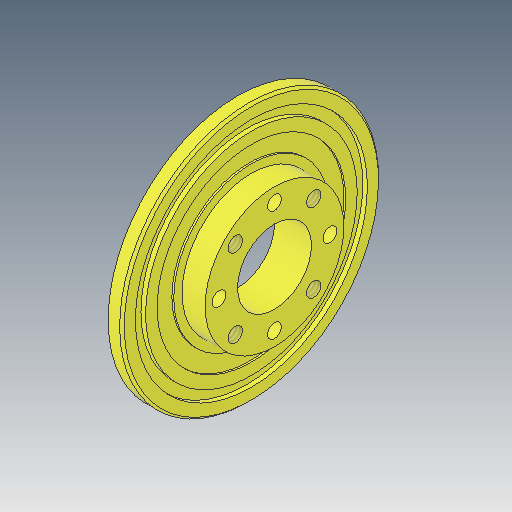
# Autodesk Inventor part: COXA_PITCH_BEARING_BASE
Saved by Autodesk Inventor 2019.4 (Build 234330000, 330)
## iProperties
Created: 2019-11-12
Part Number: COXA_PITCH_BEARING_BASE
Material: 一般
Document SubType Name: Modeling
Designer: y6tada
Density: 1 g/cm^3
Appearance: 滑らか - 黄
Mass: 1.03998 g
Surface Area: 16.9167 cm^2
Volume: 1.03998 cm^3
Author: y6tada
Autodesk Inventor part; units mm, degrees
ref_plane "YZ Plane" through (0, 0, 0) normal (1, 0, 0) x (0, 1, 0)
ref_plane "XZ Plane" through (0, 0, 0) normal (0, 1, 0) x (-1, 0, 0)
ref_plane "XY Plane" through (0, 0, 0) normal (0, 0, 1) x (1, 0, 0)
sketch "スケッチ1" plane through (0, 0, 0) normal (1, 0, 0) x (0, 1, 0)
  circle A0 centre (0, 0) radius 14
  circle A1 centre (0, 0) radius 4
  dimension "d0" = 8
  dimension "d1" = 28
  constraints: 2 centre point, 2 coincident
  measures "d0" diameter of A1
  measures "d1" diameter of A0
extrude "押し出し1" add sketch "スケッチ1" along normal blind 1.5
sketch "スケッチ2" plane through (1.5, 0, 0) normal (1, 0, 0) x (0, 0, -1)
  circle A0 centre (0, 0) radius 4 projected
  circle A1 centre (0, 0) radius 7.5
  dimension "d9" = 15
  constraints: 1 centre point, 1 coincident
  measures "d9" diameter of A1
extrude "押し出し2" add sketch "スケッチ2" along normal blind 2.5
sketch "スケッチ3" plane through (4, 0, 0) normal (1, 0, 0) x (0, 0, -1)
  circle A0 centre (0, 0) radius 6 construction
  line L0 (0, 0) -> (6, 0) construction
  point P0 (0, 6)
  point P1 (-6, 0)
  point P2 (0, -6)
  dimension "d12" = 12
  dimension "d15" = 360
  constraints: 2 end point, 1 coincident, 1 horizontal, 1 horizontal alignment, 7 other
hole "穴1" at (4, 0, -6) at (4, 6, 0) at (4, 0, 6) at (4, -6, 0) direction (-1, 0, 0) diameter 1.5 end through all both
sketch "スケッチ4" plane through (4, 0, 0) normal (1, 0, 0) x (0, 0, -1)
  line L0 (0, 0) -> (4.2426, 4.2426) construction
  circle A0 centre (0, 0) radius 6 construction
  line L1 (0, 0) -> (12.9289, 0) construction
  point P0 (-4.2426, 4.2426)
  point P1 (-4.2426, -4.2426)
  point P2 (4.2426, -4.2426)
  dimension "d25" = 12
  dimension "d24" = 45
  dimension "d28" = 360
  constraints: 4 end point, 1 coincident, 1 horizontal, 8 other
  measures "d24" angle of L1 L0
hole "穴2" at (4, 4.2426, -4.2426) at (4, 4.2426, 4.2426) at (4, -4.2426, 4.2426) at (4, -4.2426, -4.2426) direction (-1, 0, 0) diameter 1.567 end through all thread size "M2x0.4" class "6H" standard "ISO Metric profile"
sketch "スケッチ7" plane through (1.5, 0, 0) normal (1, 0, 0) x (0, 0, -1)
  circle A0 centre (0, 0) radius 8.4
  circle A1 centre (0, 0) radius 10.2
  dimension "d37" = 16.8
  dimension "d48" = 20.4
  constraints: 2 centre point, 2 coincident
  measures "d37" diameter of A0
  measures "d48" diameter of A1
extrude "押し出し3" cut sketch "スケッチ7" against normal blind 0.2
sketch "スケッチ8" plane through (1.5, 0, 0) normal (1, 0, 0) x (0, 0, -1)
  circle A0 centre (0, 0) radius 12 construction
  circle A1 centre (0, 0) radius 12.55
  circle A2 centre (0, 0) radius 11.45
  dimension "d40" = 24
  dimension "d41" = 0.55
  dimension "d42" = 0.55
  constraints: 3 centre point, 1 coincident
  measures "d40" diameter of A0
  measures "d41" radial gap between concentric circles of A0 A1
  measures "d42" radial gap between concentric circles of A2 A0
extrude "押し出し4" cut sketch "スケッチ8" against normal blind 0.5
chamfer "面取り1" distance 0.25 angle 45 1 edges at (1.5, -14, 0)
